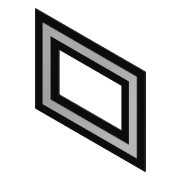
# Autodesk Inventor part: square
Saved by Autodesk Inventor 2012 (Build 160160000, 160)
## iProperties
Created: 2011-07-01
Part Number: square
Document SubType Name: Modeling
Designer: dfoster
Density: 1 g/cm^3
Material: Default
Author: dfoster
Autodesk Inventor part; units mm, degrees
ref_plane "YZ Plane" through (0, 0, 0) normal (1, 0, 0) x (0, 1, 0)
ref_plane "XZ Plane" through (0, 0, 0) normal (0, 1, 0) x (-1, 0, 0)
ref_plane "XY Plane" through (0, 0, 0) normal (0, 0, 1) x (1, 0, 0)
sketch "Sketch1" plane through (0, 0, 0) normal (0, 0, 1) x (1, 0, 0)
  line L0 (0, 0) -> (711.2, 0)
  line L1 (711.2, 0) -> (711.2, 558.8)
  line L2 (711.2, 558.8) -> (0, 558.8)
  line L3 (0, 558.8) -> (0, 0)
  line L4 (50.8, 508) -> (660.4, 508)
  line L5 (660.4, 508) -> (660.4, 50.8)
  line L6 (660.4, 50.8) -> (50.8, 50.8)
  line L7 (50.8, 50.8) -> (50.8, 508)
  line L8 (609.6, 457.2) -> (101.6, 457.2)
  line L9 (101.6, 457.2) -> (101.6, 101.6)
  line L10 (101.6, 101.6) -> (609.6, 101.6)
  line L11 (609.6, 101.6) -> (609.6, 457.2)
  line L12 (152.4, 406.4) -> (558.8, 406.4)
  line L13 (558.8, 406.4) -> (558.8, 152.4)
  line L14 (558.8, 152.4) -> (152.4, 152.4)
  line L15 (152.4, 152.4) -> (152.4, 406.4)
  dimension "d2" = 50.8
  dimension "d3" = 50.8
  dimension "d4" = 50.8
  dimension "d9" = 457.2
  dimension "d10" = 609.6
  constraints: 32 end point, 8 parallel, 4 perpendicular, 1 horizontal, 9 other
  measures "d2" distance between parallel lines of L4 L2
  measures "d3" distance between parallel lines of L8 L4
  measures "d4" distance between parallel lines of L12 L8
  measures "d9" distance of L6.end L4.start
  measures "d10" distance of L4.start L4.end
extrude "Extrusion1" add sketch "Sketch1" along normal blind 4.7752 contours L3 L2 L1 L0 | L4 L5 L6 L7 | L11 L10 L9 L8
extrude "Extrusion2" add sketch "Sketch1" along normal blind 7.9375 contours L4 L5 L6 L7
body "Solid1"
